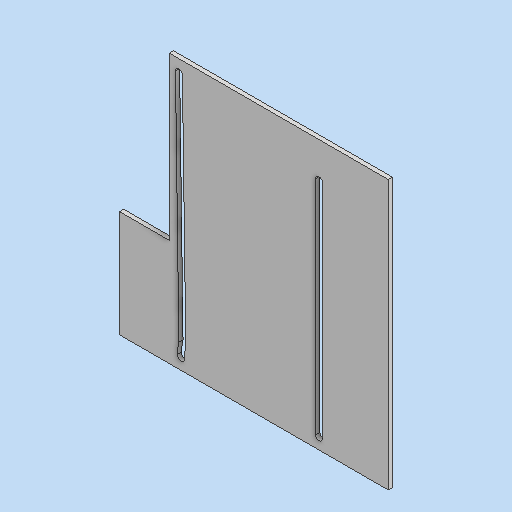
# Autodesk Inventor part: inside walls left
Saved by Autodesk Inventor 2026 (Build 300175000, 175)
## iProperties
Created: 2026-02-03
Part Number: inside walls left
Material: Generic
Document SubType Name: Modeling
Designer: mones
Density: 1 g/cm^3
Appearance: Default
Author: mones
Autodesk Inventor part; units mm, degrees
ref_plane "YZ Plane" through (0, 0, 0) normal (1, 0, 0) x (0, 1, 0)
ref_plane "XZ Plane" through (0, 0, 0) normal (0, 1, 0) x (-1, 0, 0)
ref_plane "XY Plane" through (0, 0, 0) normal (0, 0, 1) x (1, 0, 0)
sketch "Sketch1" plane through (0, 0, 0) normal (0, 0, 1) x (1, 0, 0)
  line L0 (6, 6) -> (200, 6)
  line L1 (200, 6) -> (200, 200)
  line L2 (200, 200) -> (42, 200)
  line L3 (6, 83) -> (6, 6)
  line L4 (6, 6) -> (56, 6)
  line L5 (200, 6) -> (150, 6)
  line L6 (200, 6) -> (200, 153)
  line L7 (150, 6) -> (142.5, 6)
  line L8 (200, 6) -> (200, 166)
  arc A0 (152.5, 174.3333) -> (147.5, 174.3333) centre (150, 174.3333) ccw
  line L9 (150, 6) -> (50, 6)
  arc A1 (47.8689, 14.6053) -> (52.8158, 14.5813) centre (50.3406, 14.23) ccw
  arc A2 (53.8259, 22.009) -> (52.8051, 13.8106) centre (86.918, 13.7258) ccw
  arc A3 (51.3944, 191.2047) -> (46.3962, 191.0801) centre (48.8946, 191.1682) ccw
  line L10 (53.8599, 22.4199) -> (51.3944, 191.2047)
  line L11 (48.8556, 22.7156) -> (46.3962, 191.0801)
  arc A4 (53.7373, 21.6465) -> (53.8589, 22.4929) centre (51.3599, 22.4199) ccw
  arc A5 (48.8556, 22.7156) -> (47.8689, 14.6053) centre (80.6169, 14.7362) ccw
  line L12 (52.8406, 14.23) -> (52.8088, 14.23)
  arc A6 (147.5, 14.23) -> (152.5, 14.23) centre (150, 14.23) ccw
  line L13 (147.5, 14.23) -> (147.5, 174.3333)
  line L14 (152.5, 14.23) -> (152.5, 174.3333)
  line L15 (42, 200) -> (42, 83)
  line L16 (42, 83) -> (6, 83)
  dimension "d1" = 194
  constraints: 35 end point, 20 point on circle, 7 centre point, 7 point on line, 4 tangent, 2 parallel, 2 perpendicular, 1 horizontal
  measures "d1" distance of L1.end L0.end
extrude "Extrusion1" add sketch "Sketch1" along normal blind 3
body "Solid1"
